Autodesk Inventor part; units mm, degrees
(part 4 of 10)
  spline S27 degree 5 poles (6.5254, -0.8339) (6.5255, -0.8339) (6.5256, -0.8339) (6.5259, -0.834) (6.5263, -0.834) (6.5268, -0.834) (6.5274, -0.8341) (6.5281, -0.8342) (6.5289, -0.8343) (6.5298, -0.8343) (6.5307, -0.8344) (6.5318, -0.8345) (6.5329, -0.8346) (6.5341, -0.8347) (6.5353, -0.8348) (6.5366, -0.8349) (6.5381, -0.8349) (6.5395, -0.835) (6.5411, -0.8351) (6.5427, -0.8352) (6.5444, -0.8353) (6.5462, -0.8354) (6.548, -0.8355) (6.55, -0.8356) (6.5519, -0.8356) (6.554, -0.8357) (6.5561, -0.8358) (6.5583, -0.8358) (6.5606, -0.8359) (6.5629, -0.8359) (6.5653, -0.836) (6.5678, -0.836) (6.5703, -0.836) (6.5729, -0.8361) (6.5755, -0.8361) (6.5788, -0.8361) (6.5821, -0.8361) (6.5856, -0.836) (6.5903, -0.836) (6.5964, -0.8359) (6.6022, -0.8358) (6.6081, -0.8356) (6.6149, -0.8353) (6.6206, -0.8351) (6.6249, -0.8349) (6.6293, -0.8347) (6.6352, -0.8344) (6.6406, -0.8341) (6.646, -0.8337) (6.6524, -0.8333) (6.6589, -0.8328) (6.6639, -0.8324) (6.6697, -0.832) (6.6757, -0.8314) (6.6809, -0.831) (6.6871, -0.8304) (6.6934, -0.8298) (6.6988, -0.8292) (6.7053, -0.8286) (6.7118, -0.8278) (6.7175, -0.8272) (6.7242, -0.8264) (6.731, -0.8256) (6.737, -0.8248) (6.7439, -0.8239) (6.751, -0.823) (6.7571, -0.8221) (6.7644, -0.8211) (6.7717, -0.82) (6.778, -0.8191) (6.7855, -0.8179) (6.7931, -0.8167) (6.7996, -0.8156) (6.8074, -0.8144) (6.8152, -0.813) (6.8219, -0.8118) (6.8299, -0.8104) (6.8379, -0.809) (6.8449, -0.8077) (6.8531, -0.8061) (6.8613, -0.8045) (6.8685, -0.8031) (6.8769, -0.8014) (6.8853, -0.7997) (6.8927, -0.7981) (6.9013, -0.7963) (6.91, -0.7944) (6.9175, -0.7927) (6.9263, -0.7907) (6.9352, -0.7887) (6.9428, -0.7869) (6.9519, -0.7848) (6.9609, -0.7826) (6.9688, -0.7806) (6.978, -0.7783) (6.9873, -0.776) (6.9953, -0.7739) (7.0047, -0.7715) (7.0142, -0.769) (7.0223, -0.7668) (7.0319, -0.7642) (7.0415, -0.7615) (7.0499, -0.7591) (7.0596, -0.7564) (7.0694, -0.7535) (7.0779, -0.7511) (7.0878, -0.7481) (7.0978, -0.7451) (7.1064, -0.7425) (7.1165, -0.7394) (7.1267, -0.7362) (7.1354, -0.7334) (7.1457, -0.7302) (7.156, -0.7268) (7.1649, -0.7239) (7.1753, -0.7205) (7.1857, -0.7169) (7.1947, -0.7139) (7.2053, -0.7103) (7.2159, -0.7066) (7.225, -0.7034) (7.2357, -0.6996) (7.2465, -0.6957) (7.2558, -0.6923) (7.2666, -0.6883) (7.2775, -0.6843) (7.2869, -0.6808) (7.2978, -0.6766) (7.3089, -0.6724) (7.3183, -0.6687) (7.3295, -0.6644) (7.3406, -0.66) (7.3502, -0.6561) (7.3614, -0.6516) (7.3727, -0.647) (7.3824, -0.643) (7.3937, -0.6383) (7.4051, -0.6335) (7.4149, -0.6294) (7.4264, -0.6245) (7.4379, -0.6195) (7.4478, -0.6152) (7.4594, -0.6101) (7.471, -0.605) (7.481, -0.6005) (7.4927, -0.5952) (7.5044, -0.5899) (7.5145, -0.5853) (7.5263, -0.5798) (7.5381, -0.5743) (7.5482, -0.5695) (7.5584, -0.5646) (7.5703, -0.5589) (7.5806, -0.554) (7.5908, -0.549) (7.6028, -0.5431) (7.6149, -0.5371) (7.6252, -0.5319) (7.6373, -0.5259) (7.6494, -0.5197) (7.6598, -0.5144) (7.6703, -0.509) (7.6842, -0.5017) (7.6964, -0.4953) (7.7087, -0.4888) (7.721, -0.4823) (7.7333, -0.4756) (7.7421, -0.4709) (7.7509, -0.4661) (7.7598, -0.4612) (7.7686, -0.4563) (7.7775, -0.4514) (7.7863, -0.4465) (7.7952, -0.4415) (7.8041, -0.4365) (7.813, -0.4314) (7.822, -0.4263) (7.8309, -0.4212) (7.8398, -0.4161) (7.8488, -0.4109) (7.8578, -0.4056) (7.8667, -0.4004) (7.8757, -0.3951) (7.8847, -0.3897) (7.8937, -0.3843) (7.9028, -0.3789) (7.9118, -0.3735) (7.9208, -0.368) (7.9299, -0.3625) (7.9389, -0.357) (7.9534, -0.348) (7.9662, -0.3401) (7.9771, -0.3333) (7.9862, -0.3275) (7.9935, -0.3229) knots 0 0 0 0 0 0 0.004167 0.008333 0.0125 0.016667 0.020833 0.025 0.029167 0.033333 0.0375 0.041667 0.045833 0.05 0.054167 0.058333 0.0625 0.066667 0.070833 0.075 0.079167 0.083333 0.0875 0.091667 0.095833 0.1 0.104167 0.108333 0.1125 0.116667 0.120833 0.125 0.129167 0.133333 0.1375 0.141667 0.15 0.154167 0.158333 0.170833 0.183333 0.1875 0.191667 0.2 0.204167 0.208333 0.2125 0.225 0.229167 0.233333 0.241667 0.245833 0.25 0.258333 0.2625 0.266667 0.275 0.279167 0.283333 0.291667 0.295833 0.3 0.308333 0.3125 0.316667 0.325 0.329167 0.333333 0.341667 0.345833 0.35 0.358333 0.3625 0.366667 0.375 0.379167 0.383333 0.391667 0.395833 0.4 0.408333 0.4125 0.416667 0.425 0.429167 0.433333 0.441667 0.445833 0.45 0.458333 0.4625 0.466667 0.475 0.479167 0.483333 0.491667 0.495833 0.5 0.508333 0.5125 0.516667 0.525 0.529167 0.533333 0.541667 0.545833 0.55 0.558333 0.5625 0.566667 0.575 0.579167 0.583333 0.591667 0.595833 0.6 0.608333 0.6125 0.616667 0.625 0.629167 0.633333 0.641667 0.645833 0.65 0.658333 0.6625 0.666667 0.675 0.679167 0.683333 0.691667 0.695833 0.7 0.708333 0.7125 0.716667 0.725 0.729167 0.733333 0.741667 0.745833 0.75 0.758333 0.7625 0.766667 0.775 0.779167 0.783333 0.791667 0.795833 0.8 0.804167 0.8125 0.816667 0.820833 0.829167 0.833333 0.8375 0.845833 0.85 0.854167 0.858333 0.870833 0.875 0.879167 0.883333 0.8875 0.891667 0.895833 0.9 0.904167 0.908333 0.9125 0.916667 0.920833 0.925 0.929167 0.933333 0.9375 0.941667 0.945833 0.95 0.954167 0.958333 0.9625 0.966667 0.970833 0.975 0.979167 0.983333 1 1 1 1 1 1
  line L55 (6.5248, 0.8338) -> (5.7036, 0.7289)
  point P0 (0, 0)
sketch "Block2" plane through (0, 0, 0) normal (0, 0, 1) x (1, 0, 0)
  arc A0 (-0.6063, 1.979) -> (-0.252, 3.0198) centre (-4.8955, 4.02) ccw
  line L0 (0.1956, 1.5974) -> (-0.6063, 1.979)
  line L1 (0.1962, 1.5971) -> (0.1956, 1.5974)
  spline S0 degree 5 poles (1.0882, 0.3875) (1.0858, 0.3933) (1.0826, 0.401) (1.0786, 0.4107) (1.0738, 0.4222) (1.0681, 0.4355) (1.064, 0.4451) (1.0599, 0.4545) (1.0558, 0.464) (1.0517, 0.4734) (1.0476, 0.4827) (1.0434, 0.4921) (1.0393, 0.5014) (1.0351, 0.5106) (1.0309, 0.5199) (1.0267, 0.5291) (1.0225, 0.5382) (1.0183, 0.5474) (1.0141, 0.5565) (1.0098, 0.5655) (1.0056, 0.5745) (1.0013, 0.5835) (0.997, 0.5925) (0.9928, 0.6014) (0.9885, 0.6103) (0.9841, 0.6191) (0.9798, 0.6279) (0.9755, 0.6367) (0.9711, 0.6454) (0.9668, 0.6541) (0.9616, 0.6645) (0.9563, 0.6748) (0.951, 0.6851) (0.9449, 0.6971) (0.9387, 0.7089) (0.9334, 0.719) (0.9281, 0.7291) (0.9227, 0.7391) (0.9174, 0.7491) (0.912, 0.759) (0.9067, 0.7688) (0.9004, 0.7802) (0.8941, 0.7916) (0.8887, 0.8012) (0.8824, 0.8125) (0.876, 0.8236) (0.8706, 0.8331) (0.8642, 0.8441) (0.8579, 0.855) (0.8524, 0.8643) (0.8451, 0.8766) (0.8378, 0.8889) (0.8314, 0.8995) (0.8249, 0.91) (0.8167, 0.9234) (0.8102, 0.9338) (0.8038, 0.9441) (0.7973, 0.9543) (0.789, 0.9673) (0.7826, 0.9774) (0.7761, 0.9874) (0.7687, 0.9987) (0.7613, 1.0098) (0.7557, 1.0182) (0.7492, 1.0278) (0.7428, 1.0374) (0.7372, 1.0455) (0.7307, 1.055) (0.7242, 1.0643) (0.7187, 1.0723) (0.7122, 1.0815) (0.7057, 1.0906) (0.7001, 1.0983) (0.6936, 1.1073) (0.6872, 1.1162) (0.6816, 1.1238) (0.6752, 1.1326) (0.6687, 1.1412) (0.6632, 1.1486) (0.6567, 1.1571) (0.6503, 1.1656) (0.6447, 1.1727) (0.6383, 1.1811) (0.6319, 1.1893) (0.6264, 1.1963) (0.62, 1.2043) (0.6136, 1.2123) (0.6081, 1.2191) (0.6018, 1.2269) (0.5954, 1.2347) (0.59, 1.2413) (0.5837, 1.2489) (0.5774, 1.2564) (0.572, 1.2628) (0.5657, 1.2702) (0.5594, 1.2775) (0.5541, 1.2837) (0.5479, 1.2908) (0.5416, 1.2979) (0.5363, 1.3039) (0.5302, 1.3108) (0.524, 1.3176) (0.5188, 1.3234) (0.5127, 1.3301) (0.5066, 1.3367) (0.5014, 1.3423) (0.4954, 1.3487) (0.4894, 1.3551) (0.4843, 1.3605) (0.4783, 1.3667) (0.4724, 1.3728) (0.4673, 1.378) (0.4615, 1.384) (0.4557, 1.3898) (0.4507, 1.3948) (0.4449, 1.4006) (0.4392, 1.4062) (0.4343, 1.411) (0.4286, 1.4165) (0.423, 1.4219) (0.4182, 1.4265) (0.4127, 1.4317) (0.4071, 1.4369) (0.4024, 1.4413) (0.397, 1.4463) (0.3916, 1.4512) (0.387, 1.4554) (0.3817, 1.4602) (0.3764, 1.4649) (0.372, 1.4689) (0.3668, 1.4734) (0.3617, 1.4779) (0.3573, 1.4816) (0.3523, 1.4859) (0.3473, 1.4901) (0.3431, 1.4937) (0.3382, 1.4978) (0.3333, 1.5018) (0.3293, 1.5051) (0.3245, 1.5089) (0.3199, 1.5127) (0.3159, 1.5158) (0.3114, 1.5194) (0.3069, 1.5229) (0.3031, 1.5259) (0.2988, 1.5292) (0.2945, 1.5325) (0.2908, 1.5353) (0.2867, 1.5384) (0.2826, 1.5414) (0.2791, 1.5439) (0.2752, 1.5468) (0.2713, 1.5496) (0.268, 1.552) (0.2648, 1.5542) (0.2606, 1.5572) (0.257, 1.5597) (0.253, 1.5624) (0.2491, 1.5651) (0.2453, 1.5676) (0.2426, 1.5694) (0.2399, 1.5712) (0.2377, 1.5726) (0.2356, 1.574) (0.2335, 1.5753) (0.2314, 1.5766) (0.2294, 1.5779) (0.2275, 1.5791) (0.2256, 1.5803) (0.2237, 1.5814) (0.2219, 1.5825) (0.2202, 1.5836) (0.2185, 1.5846) (0.2168, 1.5856) (0.2153, 1.5865) (0.2137, 1.5874) (0.2123, 1.5883) (0.2108, 1.5891) (0.2095, 1.5899) (0.2082, 1.5906) (0.2069, 1.5913) (0.2057, 1.592) (0.2046, 1.5926) (0.2036, 1.5932) (0.2026, 1.5938) (0.2016, 1.5943) (0.2008, 1.5947) (0.1999, 1.5952) (0.1992, 1.5955) (0.1985, 1.5959) (0.1979, 1.5962) (0.1973, 1.5965) (0.1968, 1.5968) (0.1965, 1.5969) (0.1963, 1.597) (0.1962, 1.5971) knots -1 -1 -1 -1 -1 -1 -0.9875 -0.983333 -0.979167 -0.975 -0.970833 -0.966667 -0.9625 -0.958333 -0.954167 -0.95 -0.945833 -0.941667 -0.9375 -0.933333 -0.929167 -0.925 -0.920833 -0.916667 -0.9125 -0.908333 -0.904167 -0.9 -0.895833 -0.891667 -0.8875 -0.883333 -0.879167 -0.875 -0.870833 -0.8625 -0.858333 -0.854167 -0.845833 -0.841667 -0.8375 -0.833333 -0.829167 -0.820833 -0.816667 -0.8125 -0.804167 -0.8 -0.795833 -0.7875 -0.783333 -0.779167 -0.770833 -0.766667 -0.7625 -0.75 -0.745833 -0.741667 -0.7375 -0.725 -0.720833 -0.716667 -0.7125 -0.7 -0.695833 -0.691667 -0.683333 -0.679167 -0.675 -0.666667 -0.6625 -0.658333 -0.65 -0.645833 -0.641667 -0.633333 -0.629167 -0.625 -0.616667 -0.6125 -0.608333 -0.6 -0.595833 -0.591667 -0.583333 -0.579167 -0.575 -0.566667 -0.5625 -0.558333 -0.55 -0.545833 -0.541667 -0.533333 -0.529167 -0.525 -0.516667 -0.5125 -0.508333 -0.5 -0.495833 -0.491667 -0.483333 -0.479167 -0.475 -0.466667 -0.4625 -0.458333 -0.45 -0.445833 -0.441667 -0.433333 -0.429167 -0.425 -0.416667 -0.4125 -0.408333 -0.4 -0.395833 -0.391667 -0.383333 -0.379167 -0.375 -0.366667 -0.3625 -0.358333 -0.35 -0.345833 -0.341667 -0.333333 -0.329167 -0.325 -0.316667 -0.3125 -0.308333 -0.3 -0.295833 -0.291667 -0.283333 -0.279167 -0.275 -0.266667 -0.2625 -0.258333 -0.25 -0.245833 -0.241667 -0.233333 -0.229167 -0.225 -0.216667 -0.2125 -0.208333 -0.2 -0.195833 -0.191667 -0.183333 -0.179167 -0.175 -0.170833 -0.158333 -0.154167 -0.145833 -0.141667 -0.1375 -0.133333 -0.129167 -0.125 -0.120833 -0.116667 -0.1125 -0.108333 -0.104167 -0.1 -0.095833 -0.091667 -0.0875 -0.083333 -0.079167 -0.075 -0.070833 -0.066667 -0.0625 -0.058333 -0.054167 -0.05 -0.045833 -0.041667 -0.0375 -0.033333 -0.029167 -0.025 -0.020833 -0.016667 -0.0125 -0.008333 0 0 0 0 0 0
  arc A1 (0.7429, -0.1283) -> (1.0882, 0.3875) centre (-4.8955, 4.02) ccw
  line L2 (-0.7158, 0.236) -> (-0.7153, 0.2355)
  spline S1 degree 5 poles (-0.7153, 0.2355) (-0.7153, 0.2355) (-0.7152, 0.2354) (-0.715, 0.2353) (-0.7147, 0.235) (-0.7143, 0.2347) (-0.7139, 0.2343) (-0.7133, 0.2338) (-0.7128, 0.2334) (-0.7121, 0.2328) (-0.7114, 0.2322) (-0.7106, 0.2316) (-0.7098, 0.2309) (-0.7089, 0.2302) (-0.708, 0.2295) (-0.707, 0.2287) (-0.7059, 0.2278) (-0.7048, 0.2269) (-0.7036, 0.226) (-0.7024, 0.2251) (-0.7011, 0.2241) (-0.6997, 0.223) (-0.6983, 0.2219) (-0.6968, 0.2208) (-0.6953, 0.2197) (-0.6937, 0.2185) (-0.6921, 0.2173) (-0.6904, 0.2161) (-0.6886, 0.2148) (-0.6868, 0.2135) (-0.6849, 0.2121) (-0.683, 0.2108) (-0.6806, 0.2091) (-0.6781, 0.2074) (-0.6756, 0.2056) (-0.6725, 0.2035) (-0.6693, 0.2014) (-0.6665, 0.1995) (-0.6631, 0.1972) (-0.6596, 0.1949) (-0.6565, 0.1929) (-0.6534, 0.1909) (-0.6496, 0.1885) (-0.6446, 0.1853) (-0.6394, 0.1821) (-0.634, 0.1788) (-0.6285, 0.1754) (-0.6227, 0.172) (-0.6182, 0.1693) (-0.6135, 0.1666) (-0.6088, 0.1638) (-0.6032, 0.1606) (-0.5982, 0.1578) (-0.5938, 0.1554) (-0.5887, 0.1525) (-0.5834, 0.1497) (-0.5788, 0.1472) (-0.5734, 0.1442) (-0.5678, 0.1413) (-0.563, 0.1387) (-0.5572, 0.1358) (-0.5514, 0.1328) (-0.5463, 0.1302) (-0.5403, 0.1271) (-0.5342, 0.1241) (-0.5289, 0.1215) (-0.5226, 0.1184) (-0.5162, 0.1153) (-0.5107, 0.1127) (-0.5041, 0.1096) (-0.4975, 0.1065) (-0.4917, 0.1038) (-0.4849, 0.1007) (-0.478, 0.0975) (-0.472, 0.0949) (-0.4649, 0.0917) (-0.4577, 0.0886) (-0.4515, 0.0859) (-0.4442, 0.0827) (-0.4367, 0.0796) (-0.4303, 0.0769) (-0.4227, 0.0737) (-0.415, 0.0706) (-0.4083, 0.0679) (-0.4005, 0.0647) (-0.3925, 0.0616) (-0.3856, 0.0589) (-0.3775, 0.0558) (-0.3693, 0.0527) (-0.3623, 0.05) (-0.3539, 0.0469) (-0.3455, 0.0438) (-0.3382, 0.0411) (-0.3296, 0.038) (-0.3209, 0.035) (-0.3134, 0.0323) (-0.3045, 0.0293) (-0.2956, 0.0262) (-0.2879, 0.0237) (-0.2788, 0.0206) (-0.2697, 0.0176) (-0.2618, 0.0151) (-0.2525, 0.0121) (-0.2431, 0.0091) (-0.235, 0.0066) (-0.2254, 0.0037) (-0.2158, 0.0008) (-0.2075, -0.0017) (-0.1977, -0.0046) (-0.1879, -0.0074) (-0.1794, -0.0099) (-0.1694, -0.0127) (-0.1593, -0.0155) (-0.1506, -0.0179) (-0.1404, -0.0206) (-0.1301, -0.0234) (-0.1213, -0.0257) (-0.1108, -0.0284) (-0.1003, -0.031) (-0.0913, -0.0333) (-0.0806, -0.0359) (-0.0699, -0.0385) (-0.0606, -0.0407) (-0.0498, -0.0432) (-0.0389, -0.0457) (-0.0294, -0.0479) (-0.0184, -0.0503) (-0.0072, -0.0528) (0.0024, -0.0548) (0.0136, -0.0572) (0.025, -0.0595) (0.0347, -0.0615) (0.0462, -0.0638) (0.0578, -0.0661) (0.0677, -0.068) (0.0794, -0.0701) (0.0911, -0.0723) (0.1012, -0.0741) (0.1131, -0.0762) (0.125, -0.0783) (0.1353, -0.08) (0.1474, -0.082) (0.1595, -0.084) (0.1699, -0.0856) (0.1822, -0.0875) (0.1945, -0.0894) (0.2051, -0.0909) (0.2193, -0.0929) (0.2336, -0.0949) (0.2462, -0.0966) (0.2589, -0.0983) (0.2716, -0.0999) (0.2862, -0.1017) (0.3008, -0.1034) (0.3156, -0.1051) (0.3305, -0.1067) (0.3473, -0.1085) (0.3585, -0.1096) (0.3698, -0.1108) (0.3849, -0.1122) (0.4002, -0.1136) (0.4135, -0.1147) (0.427, -0.1158) (0.4405, -0.1169) (0.4501, -0.1176) (0.4598, -0.1183) (0.4696, -0.119) (0.4793, -0.1197) (0.4891, -0.1203) (0.4989, -0.1209) (0.5088, -0.1215) (0.5187, -0.1221) (0.5286, -0.1226) (0.5385, -0.1232) (0.5485, -0.1237) (0.5584, -0.1241) (0.5685, -0.1246) (0.5785, -0.125) (0.5886, -0.1254) (0.5987, -0.1258) (0.6088, -0.1261) (0.619, -0.1264) (0.6291, -0.1267) (0.6394, -0.127) (0.6496, -0.1272) (0.6599, -0.1275) (0.6701, -0.1277) (0.6805, -0.1278) (0.6908, -0.128) (0.7053, -0.1281) (0.7178, -0.1282) (0.7283, -0.1283) (0.7366, -0.1283) (0.7429, -0.1283) knots 0 0 0 0 0 0 0.004167 0.008333 0.0125 0.016667 0.020833 0.025 0.029167 0.033333 0.0375 0.041667 0.045833 0.05 0.054167 0.058333 0.0625 0.066667 0.070833 0.075 0.079167 0.083333 0.0875 0.091667 0.095833 0.1 0.104167 0.108333 0.1125 0.116667 0.120833 0.125 0.129167 0.1375 0.141667 0.145833 0.154167 0.158333 0.1625 0.170833 0.175 0.179167 0.183333 0.191667 0.208333 0.2125 0.216667 0.220833 0.229167 0.2375 0.241667 0.245833 0.254167 0.258333 0.2625 0.270833 0.275 0.279167 0.2875 0.291667 0.295833 0.304167 0.308333 0.3125 0.320833 0.325 0.329167 0.3375 0.341667 0.345833 0.354167 0.358333 0.3625 0.370833 0.375 0.379167 0.3875 0.391667 0.395833 0.404167 0.408333 0.4125 0.420833 0.425 0.429167 0.4375 0.441667 0.445833 0.454167 0.458333 0.4625 0.470833 0.475 0.479167 0.4875 0.491667 0.495833 0.504167 0.508333 0.5125 0.520833 0.525 0.529167 0.5375 0.541667 0.545833 0.554167 0.558333 0.5625 0.570833 0.575 0.579167 0.5875 0.591667 0.595833 0.604167 0.608333 0.6125 0.620833 0.625 0.629167 0.6375 0.641667 0.645833 0.654167 0.658333 0.6625 0.670833 0.675 0.679167 0.6875 0.691667 0.695833 0.704167 0.708333 0.7125 0.720833 0.725 0.729167 0.7375 0.741667 0.745833 0.754167 0.758333 0.7625 0.770833 0.775 0.779167 0.791667 0.795833 0.8 0.804167 0.808333 0.825 0.829167 0.833333 0.8375 0.845833 0.85 0.854167 0.866667 0.870833 0.875 0.879167 0.883333 0.8875 0.891667 0.895833 0.9 0.904167 0.908333 0.9125 0.916667 0.920833 0.925 0.929167 0.933333 0.9375 0.941667 0.945833 0.95 0.954167 0.958333 0.9625 0.966667 0.970833 0.975 0.979167 0.983333 0.9875 1 1 1 1 1 1
  line L3 (-1.3742, 0.832) -> (-0.7158, 0.236)
  arc A2 (-2.2015, 0.1079) -> (-1.3742, 0.832) centre (-4.8955, 4.02) ccw
  line L4 (0.6162, 2.8328) -> (0.6169, 2.8327)
  line L5 (-0.252, 3.0198) -> (0.6162, 2.8328)
  spline S2 degree 5 poles (0.6169, 2.8327) (0.6169, 2.8326) (0.6171, 2.8326) (0.6173, 2.8326) (0.6176, 2.8325) (0.6182, 2.8324) (0.6188, 2.8323) (0.6194, 2.8322) (0.6202, 2.832) (0.621, 2.8319) (0.6219, 2.8317) (0.6229, 2.8316) (0.6239, 2.8314) (0.6251, 2.8312) (0.6263, 2.831) (0.6275, 2.8309) (0.6289, 2.8307) (0.6303, 2.8305) (0.6318, 2.8302) (0.6333, 2.83) (0.6349, 2.8298) (0.6366, 2.8296) (0.6384, 2.8294) (0.6402, 2.8292) (0.6421, 2.8289) (0.6441, 2.8287) (0.6461, 2.8285) (0.6482, 2.8283) (0.6504, 2.828) (0.6526, 2.8278) (0.6549, 2.8276) (0.6572, 2.8274) (0.6601, 2.8271) (0.6631, 2.8269) (0.6662, 2.8266) (0.67, 2.8263) (0.6738, 2.826) (0.6772, 2.8258) (0.6812, 2.8256) (0.6854, 2.8253) (0.6891, 2.8251) (0.6935, 2.8249) (0.698, 2.8247) (0.7019, 2.8246) (0.7066, 2.8244) (0.7115, 2.8243) (0.7157, 2.8241) (0.7207, 2.824) (0.7258, 2.824) (0.7303, 2.8239) (0.7356, 2.8239) (0.7411, 2.8238) (0.7458, 2.8238) (0.7514, 2.8239) (0.7572, 2.8239) (0.7621, 2.824) (0.768, 2.8241) (0.774, 2.8242) (0.7793, 2.8244) (0.7855, 2.8246) (0.7917, 2.8248) (0.7972, 2.825) (0.8037, 2.8253) (0.8102, 2.8256) (0.8159, 2.8259) (0.8226, 2.8263) (0.8294, 2.8267) (0.8353, 2.8271) (0.8423, 2.8276) (0.8494, 2.8281) (0.8555, 2.8286) (0.8627, 2.8291) (0.87, 2.8298) (0.8764, 2.8304) (0.8839, 2.8311) (0.8914, 2.8318) (0.8979, 2.8325) (0.9056, 2.8333) (0.9134, 2.8342) (0.9202, 2.8349) (0.9281, 2.8359) (0.9361, 2.8369) (0.9431, 2.8378) (0.9512, 2.8388) (0.9594, 2.84) (0.9666, 2.841) (0.9749, 2.8422) (0.9834, 2.8434) (0.9907, 2.8445) (0.9993, 2.8459) (1.0079, 2.8473) (1.0154, 2.8485) (1.0242, 2.85) (1.033, 2.8515) (1.0407, 2.8529) (1.0497, 2.8545) (1.0587, 2.8562) (1.0666, 2.8577) (1.0757, 2.8594) (1.085, 2.8612) (1.093, 2.8629) (1.1023, 2.8648) (1.1118, 2.8668) (1.1199, 2.8685) (1.1294, 2.8706) (1.1391, 2.8727) (1.1473, 2.8746) (1.1571, 2.8768) (1.1668, 2.8791) (1.1753, 2.8811) (1.1852, 2.8835) (1.1951, 2.8859) (1.2037, 2.8881) (1.2138, 2.8906) (1.2239, 2.8932) (1.2326, 2.8955) (1.2428, 2.8983) (1.2531, 2.901) (1.2619, 2.9035) (1.2723, 2.9063) (1.2828, 2.9093) (1.2917, 2.9119) (1.3023, 2.9149) (1.3128, 2.918) (1.3219, 2.9208) (1.3326, 2.924) (1.3433, 2.9273) (1.3526, 2.9301) (1.3634, 2.9335) (1.3742, 2.937) (1.3836, 2.94) (1.3945, 2.9436) (1.4055, 2.9473) (1.415, 2.9504) (1.426, 2.9542) (1.4372, 2.958) (1.4467, 2.9613) (1.4579, 2.9653) (1.4692, 2.9693) (1.4789, 2.9727) (1.4902, 2.9769) (1.5015, 2.9811) (1.5113, 2.9847) (1.5228, 2.989) (1.5342, 2.9934) (1.5441, 2.9972) (1.5557, 3.0016) (1.5672, 3.0062) (1.5772, 3.0102) (1.5872, 3.0142) (1.6022, 3.0202) (1.6157, 3.0257) (1.6291, 3.0313) (1.6426, 3.037) (1.6596, 3.0443) (1.6715, 3.0494) (1.6834, 3.0546) (1.6954, 3.0599) (1.7108, 3.0668) (1.7229, 3.0722) (1.7349, 3.0777) (1.7488, 3.084) (1.7627, 3.0905) (1.7731, 3.0954) (1.7835, 3.1003) (1.794, 3.1053) (1.8028, 3.1095) (1.8115, 3.1138) (1.8203, 3.118) (1.8291, 3.1223) (1.8379, 3.1267) (1.8467, 3.1311) (1.8555, 3.1355) (1.8643, 3.1399) (1.8732, 3.1444) (1.882, 3.1489) (1.8909, 3.1535) (1.8998, 3.1581) (1.9087, 3.1627) (1.9176, 3.1673) (1.9265, 3.172) (1.9355, 3.1768) (1.9444, 3.1815) (1.9534, 3.1863) (1.9623, 3.1911) (1.9713, 3.196) (1.9803, 3.2009) (1.9893, 3.2059) (1.9983, 3.2108) (2.0073, 3.2159) (2.0164, 3.2209) (2.029, 3.228) (2.0399, 3.2342) (2.0489, 3.2394) (2.0562, 3.2435) (2.0617, 3.2467) knots 0 0 0 0 0 0 0.004167 0.008333 0.0125 0.016667 0.020833 0.025 0.029167 0.033333 0.0375 0.041667 0.045833 0.05 0.054167 0.058333 0.0625 0.066667 0.070833 0.075 0.079167 0.083333 0.0875 0.091667 0.095833 0.1 0.104167 0.108333 0.1125 0.116667 0.120833 0.125 0.129167 0.1375 0.141667 0.145833 0.154167 0.158333 0.1625 0.170833 0.175 0.179167 0.1875 0.191667 0.195833 0.204167 0.208333 0.2125 0.220833 0.225 0.229167 0.2375 0.241667 0.245833 0.254167 0.258333 0.2625 0.270833 0.275 0.279167 0.2875 0.291667 0.295833 0.304167 0.308333 0.3125 0.320833 0.325 0.329167 0.3375 0.341667 0.345833 0.354167 0.358333 0.3625 0.370833 0.375 0.379167 0.3875 0.391667 0.395833 0.404167 0.408333 0.4125 0.420833 0.425 0.429167 0.4375 0.441667 0.445833 0.454167 0.458333 0.4625 0.470833 0.475 0.479167 0.4875 0.491667 0.495833 0.504167 0.508333 0.5125 0.520833 0.525 0.529167 0.5375 0.541667 0.545833 0.554167 0.558333 0.5625 0.570833 0.575 0.579167 0.5875 0.591667 0.595833 0.604167 0.608333 0.6125 0.620833 0.625 0.629167 0.6375 0.641667 0.645833 0.654167 0.658333 0.6625 0.670833 0.675 0.679167 0.6875 0.691667 0.695833 0.704167 0.708333 0.7125 0.720833 0.725 0.729167 0.7375 0.741667 0.745833 0.754167 0.758333 0.7625 0.770833 0.775 0.779167 0.783333 0.8 0.804167 0.808333 0.8125 0.825 0.829167 0.833333 0.8375 0.85 0.854167 0.858333 0.866667 0.870833 0.875 0.879167 0.883333 0.8875 0.891667 0.895833 0.9 0.904167 0.908333 0.9125 0.916667 0.920833 0.925 0.929167 0.933333 0.9375 0.941667 0.945833 0.95 0.954167 0.958333 0.9625 0.966667 0.970833 0.975 0.979167 0.983333 0.9875 1 1 1 1 1 1
  line L6 (0.7249, 4.4675) -> (-0.1605, 4.397)
  line L7 (0.7255, 4.4675) -> (0.7249, 4.4675)
  arc A3 (-0.1605, 4.397) -> (-0.374, 5.4756) centre (-4.8955, 4.02) ccw
  spline S3 degree 5 poles (2.1028, 3.866) (2.0978, 3.8698) (2.0912, 3.8749) (2.0829, 3.8813) (2.0729, 3.8888) (2.0613, 3.8976) (2.053, 3.9038) (2.0448, 3.9099) (2.0365, 3.916) (2.0282, 3.9221) (2.02, 3.9282) (2.0117, 3.9342) (2.0035, 3.9402) (1.9952, 3.9461) (1.987, 3.952) (1.9788, 3.9579) (1.9705, 3.9637) (1.9623, 3.9695) (1.9541, 3.9753) (1.9459, 3.981) (1.9377, 3.9867) (1.9295, 3.9923) (1.9213, 3.9979) (1.9132, 4.0035) (1.905, 4.0091) (1.8969, 4.0146) (1.8887, 4.02) (1.8806, 4.0255) (1.8724, 4.0308) (1.8643, 4.0362) (1.8546, 4.0426) (1.8449, 4.0489) (1.8352, 4.0552) (1.8239, 4.0625) (1.8126, 4.0696) (1.8029, 4.0757) (1.7933, 4.0818) (1.7837, 4.0878) (1.7741, 4.0937) (1.7645, 4.0996) (1.7549, 4.1055) (1.7438, 4.1122) (1.7326, 4.1189) (1.7231, 4.1246) (1.712, 4.1311) (1.701, 4.1376) (1.6915, 4.1431) (1.6805, 4.1494) (1.6696, 4.1557) (1.6602, 4.161) (1.6492, 4.1672) (1.6383, 4.1733) (1.629, 4.1784) (1.6166, 4.1852) (1.6043, 4.1919) (1.5935, 4.1977) (1.5828, 4.2034) (1.569, 4.2107) (1.5583, 4.2162) (1.5477, 4.2217) (1.5371, 4.2271) (1.5235, 4.234) (1.513, 4.2393) (1.5025, 4.2445) (1.4906, 4.2504) (1.4787, 4.2561) (1.4698, 4.2604) (1.4594, 4.2653) (1.4492, 4.2702) (1.4404, 4.2743) (1.4301, 4.279) (1.42, 4.2836) (1.4113, 4.2876) (1.4012, 4.2921) (1.3911, 4.2966) (1.3825, 4.3004) (1.3725, 4.3047) (1.3626, 4.309) (1.3541, 4.3126) (1.3443, 4.3168) (1.3345, 4.3209) (1.3261, 4.3243) (1.3164, 4.3283) (1.3067, 4.3322) (1.2985, 4.3355) (1.2889, 4.3393) (1.2794, 4.343) (1.2712, 4.3462) (1.2618, 4.3498) (1.2524, 4.3533) (1.2444, 4.3563) (1.2351, 4.3597) (1.2259, 4.3631) (1.2181, 4.3659) (1.2089, 4.3692) (1.1999, 4.3724) (1.1921, 4.3751) (1.1832, 4.3781) (1.1743, 4.3812) (1.1667, 4.3837) (1.1579, 4.3866) (1.1491, 4.3894) (1.1417, 4.3918) (1.1331, 4.3946) (1.1245, 4.3972) (1.1172, 4.3995) (1.1088, 4.4021) (1.1004, 4.4046) (1.0933, 4.4067) (1.085, 4.4091) (1.0768, 4.4114) (1.0699, 4.4134) (1.0618, 4.4156) (1.0538, 4.4178) (1.047, 4.4196) (1.0391, 4.4217) (1.0314, 4.4237) (1.0247, 4.4254) (1.0171, 4.4274) (1.0095, 4.4292) (1.0031, 4.4308) (0.9956, 4.4326) (0.9883, 4.4343) (0.982, 4.4357) (0.9748, 4.4374) (0.9676, 4.4389) (0.9616, 4.4403) (0.9546, 4.4417) (0.9477, 4.4432) (0.9418, 4.4444) (0.9351, 4.4457) (0.9284, 4.447) (0.9227, 4.4481) (0.9162, 4.4493) (0.9098, 4.4505) (0.9044, 4.4514) (0.8981, 4.4525) (0.8919, 4.4536) (0.8867, 4.4544) (0.8807, 4.4554) (0.8748, 4.4563) (0.8698, 4.457) (0.8641, 4.4579) (0.8584, 4.4587) (0.8537, 4.4593) (0.8482, 4.4601) (0.8429, 4.4608) (0.8384, 4.4613) (0.8332, 4.4619) (0.8281, 4.4625) (0.8239, 4.463) (0.819, 4.4635) (0.8142, 4.464) (0.8102, 4.4644) (0.8063, 4.4647) (0.8012, 4.4652) (0.7968, 4.4656) (0.792, 4.4659) (0.7873, 4.4663) (0.7828, 4.4666) (0.7795, 4.4668) (0.7763, 4.467) (0.7737, 4.4671) (0.7711, 4.4672) (0.7686, 4.4673) (0.7662, 4.4674) (0.7639, 4.4675) (0.7616, 4.4676) (0.7593, 4.4677) (0.7571, 4.4678) (0.755, 4.4678) (0.753, 4.4679) (0.751, 4.4679) (0.7491, 4.4679) (0.7473, 4.4679) (0.7455, 4.468) (0.7438, 4.468) (0.7421, 4.468) (0.7406, 4.468) (0.7391, 4.468) (0.7377, 4.4679) (0.7363, 4.4679) (0.735, 4.4679) (0.7338, 4.4679) (0.7327, 4.4678) (0.7316, 4.4678) (0.7306, 4.4678) (0.7297, 4.4677) (0.7289, 4.4677) (0.7281, 4.4677) (0.7274, 4.4676) (0.7267, 4.4676) (0.7262, 4.4676) (0.7259, 4.4676) (0.7256, 4.4676) (0.7255, 4.4675) knots -1 -1 -1 -1 -1 -1 -0.9875 -0.983333 -0.979167 -0.975 -0.970833 -0.966667 -0.9625 -0.958333 -0.954167 -0.95 -0.945833 -0.941667 -0.9375 -0.933333 -0.929167 -0.925 -0.920833 -0.916667 -0.9125 -0.908333 -0.904167 -0.9 -0.895833 -0.891667 -0.8875 -0.883333 -0.879167 -0.875 -0.870833 -0.8625 -0.858333 -0.854167 -0.845833 -0.841667 -0.8375 -0.833333 -0.829167 -0.820833 -0.816667 -0.8125 -0.804167 -0.8 -0.795833 -0.7875 -0.783333 -0.779167 -0.770833 -0.766667 -0.7625 -0.754167 -0.75 -0.745833 -0.733333 -0.729167 -0.725 -0.720833 -0.708333 -0.704167 -0.7 -0.695833 -0.683333 -0.679167 -0.675 -0.666667 -0.6625 -0.658333 -0.65 -0.645833 -0.641667 -0.633333 -0.629167 -0.625 -0.616667 -0.6125 -0.608333 -0.6 -0.595833 -0.591667 -0.583333 -0.579167 -0.575 -0.566667 -0.5625 -0.558333 -0.55 -0.545833 -0.541667 -0.533333 -0.529167 -0.525 -0.516667 -0.5125 -0.508333 -0.5 -0.495833 -0.491667 -0.483333 -0.479167 -0.475 -0.466667 -0.4625 -0.458333 -0.45 -0.445833 -0.441667 -0.433333 -0.429167 -0.425 -0.416667 -0.4125 -0.408333 -0.4 -0.395833 -0.391667 -0.383333 -0.379167 -0.375 -0.366667 -0.3625 -0.358333 -0.35 -0.345833 -0.341667 -0.333333 -0.329167 -0.325 -0.316667 -0.3125 -0.308333 -0.3 -0.295833 -0.291667 -0.283333 -0.279167 -0.275 -0.266667 -0.2625 -0.258333 -0.25 -0.245833 -0.241667 -0.233333 -0.229167 -0.225 -0.216667 -0.2125 -0.208333 -0.2 -0.195833 -0.191667 -0.183333 -0.179167 -0.175 -0.170833 -0.158333 -0.154167 -0.145833 -0.141667 -0.1375 -0.133333 -0.129167 -0.125 -0.120833 -0.116667 -0.1125 -0.108333 -0.104167 -0.1 -0.095833 -0.091667 -0.0875 -0.083333 -0.079167 -0.075 -0.070833 -0.066667 -0.0625 -0.058333 -0.054167 -0.05 -0.045833 -0.041667 -0.0375 -0.033333 -0.029167 -0.025 -0.020833 -0.016667 -0.0125 -0.008333 0 0 0 0 0 0
  arc A4 (2.0617, 3.2467) -> (2.1028, 3.866) centre (-4.8955, 4.02) ccw
  line L8 (-10.4072, 5.2072) -> (-10.4079, 5.2073)
  line L9 (-9.539, 5.0202) -> (-10.4072, 5.2072)
  spline S4 degree 5 poles (-10.4079, 5.2073) (-10.4079, 5.2073) (-10.4081, 5.2073) (-10.4083, 5.2074) (-10.4086, 5.2075) (-10.4092, 5.2076) (-10.4098, 5.2077) (-10.4104, 5.2078) (-10.4112, 5.2079) (-10.412, 5.2081) (-10.4129, 5.2082) (-10.4139, 5.2084) (-10.4149, 5.2086) (-10.4161, 5.2087) (-10.4173, 5.2089) (-10.4185, 5.2091) (-10.4199, 5.2093) (-10.4213, 5.2095) (-10.4228, 5.2097) (-10.4243, 5.2099) (-10.4259, 5.2101) (-10.4276, 5.2104) (-10.4294, 5.2106) (-10.4312, 5.2108) (-10.4331, 5.211) (-10.4351, 5.2113) (-10.4371, 5.2115) (-10.4392, 5.2117) (-10.4414, 5.2119) (-10.4436, 5.2122) (-10.4459, 5.2124) (-10.4482, 5.2126) (-10.4511, 5.2129) (-10.4541, 5.2131) (-10.4572, 5.2134) (-10.461, 5.2136) (-10.4648, 5.2139) (-10.4682, 5.2141) (-10.4722, 5.2144) (-10.4764, 5.2146) (-10.4801, 5.2148) (-10.4845, 5.215) (-10.489, 5.2152) (-10.4929, 5.2154) (-10.4976, 5.2156) (-10.5025, 5.2157) (-10.5067, 5.2158) (-10.5117, 5.2159) (-10.5168, 5.216) (-10.5213, 5.2161) (-10.5266, 5.2161) (-10.5321, 5.2161) (-10.5368, 5.2161) (-10.5424, 5.2161) (-10.5482, 5.2161) (-10.5531, 5.216) (-10.559, 5.2159) (-10.565, 5.2157) (-10.5703, 5.2156) (-10.5765, 5.2154) (-10.5827, 5.2152) (-10.5882, 5.215) (-10.5947, 5.2147) (-10.6012, 5.2144) (-10.6069, 5.2141) (-10.6136, 5.2137) (-10.6204, 5.2133) (-10.6263, 5.2129) (-10.6333, 5.2124) (-10.6404, 5.2119) (-10.6465, 5.2114) (-10.6537, 5.2108) (-10.661, 5.2102) (-10.6674, 5.2096) (-10.6749, 5.2089) (-10.6824, 5.2082) (-10.6889, 5.2075) (-10.6966, 5.2067) (-10.7044, 5.2058) (-10.7112, 5.205) (-10.7191, 5.2041) (-10.7271, 5.2031) (-10.7341, 5.2022) (-10.7422, 5.2011) (-10.7504, 5.2) (-10.7576, 5.199) (-10.7659, 5.1978) (-10.7744, 5.1965) (-10.7817, 5.1954) (-10.7903, 5.1941) (-10.7989, 5.1927) (-10.8064, 5.1915) (-10.8152, 5.19) (-10.824, 5.1885) (-10.8317, 5.1871) (-10.8407, 5.1855) (-10.8497, 5.1838) (-10.8576, 5.1823) (-10.8667, 5.1805) (-10.876, 5.1787) (-10.884, 5.1771) (-10.8933, 5.1752) (-10.9028, 5.1732) (-10.9109, 5.1715) (-10.9204, 5.1694) (-10.9301, 5.1673) (-10.9383, 5.1654) (-10.9481, 5.1632) (-10.9578, 5.1609) (-10.9663, 5.1589) (-10.9762, 5.1565) (-10.9861, 5.154) (-10.9947, 5.1519) (-11.0048, 5.1493) (-11.0149, 5.1467) (-11.0236, 5.1444) (-11.0338, 5.1417) (-11.0441, 5.1389) (-11.0529, 5.1365) (-11.0633, 5.1336) (-11.0738, 5.1307) (-11.0827, 5.1281) (-11.0933, 5.125) (-11.1038, 5.1219) (-11.1129, 5.1192) (-11.1236, 5.116) (-11.1343, 5.1127) (-11.1436, 5.1098) (-11.1544, 5.1064) (-11.1652, 5.103) (-11.1746, 5.0999) (-11.1855, 5.0964) (-11.1965, 5.0927) (-11.206, 5.0895) (-11.217, 5.0858) (-11.2282, 5.082) (-11.2377, 5.0786) (-11.2489, 5.0747) (-11.2602, 5.0707) (-11.2699, 5.0672) (-11.2812, 5.0631) (-11.2925, 5.0589) (-11.3023, 5.0553) (-11.3138, 5.051) (-11.3252, 5.0466) (-11.3351, 5.0428) (-11.3467, 5.0383) (-11.3582, 5.0338) (-11.3682, 5.0298) (-11.3782, 5.0258) (-11.3932, 5.0197) (-11.4067, 5.0142) (-11.4201, 5.0086) (-11.4336, 5.0029) (-11.4506, 4.9957) (-11.4625, 4.9906) (-11.4744, 4.9854) (-11.4864, 4.9801) (-11.5018, 4.9732) (-11.5139, 4.9678) (-11.5259, 4.9623) (-11.5398, 4.9559) (-11.5537, 4.9495) (-11.5641, 4.9446) (-11.5745, 4.9396) (-11.585, 4.9346) (-11.5938, 4.9304) (-11.6025, 4.9262) (-11.6113, 4.9219) (-11.6201, 4.9176) (-11.6289, 4.9133) (-11.6377, 4.9089) (-11.6465, 4.9045) (-11.6553, 4.9) (-11.6642, 4.8956) (-11.673, 4.8911) (-11.6819, 4.8865) (-11.6908, 4.8819) (-11.6997, 4.8773) (-11.7086, 4.8726) (-11.7175, 4.8679) (-11.7265, 4.8632) (-11.7354, 4.8585) (-11.7444, 4.8537) (-11.7533, 4.8488) (-11.7623, 4.844) (-11.7713, 4.839) (-11.7803, 4.8341) (-11.7893, 4.8291) (-11.7983, 4.8241) (-11.8074, 4.8191) (-11.82, 4.812) (-11.8309, 4.8058) (-11.8399, 4.8006) (-11.8472, 4.7964) (-11.8527, 4.7933) knots 0 0 0 0 0 0 0.004167 0.008333 0.0125 0.016667 0.020833 0.025 0.029167 0.033333 0.0375 0.041667 0.045833 0.05 0.054167 0.058333 0.0625 0.066667 0.070833 0.075 0.079167 0.083333 0.0875 0.091667 0.095833 0.1 0.104167 0.108333 0.1125 0.116667 0.120833 0.125 0.129167 0.1375 0.141667 0.145833 0.154167 0.158333 0.1625 0.170833 0.175 0.179167 0.1875 0.191667 0.195833 0.204167 0.208333 0.2125 0.220833 0.225 0.229167 0.2375 0.241667 0.245833 0.254167 0.258333 0.2625 0.270833 0.275 0.279167 0.2875 0.291667 0.295833 0.304167 0.308333 0.3125 0.320833 0.325 0.329167 0.3375 0.341667 0.345833 0.354167 0.358333 0.3625 0.370833 0.375 0.379167 0.3875 0.391667 0.395833 0.404167 0.408333 0.4125 0.420833 0.425 0.429167 0.4375 0.441667 0.445833 0.454167 0.458333 0.4625 0.470833 0.475 0.479167 0.4875 0.491667 0.495833 0.504167 0.508333 0.5125 0.520833 0.525 0.529167 0.5375 0.541667 0.545833 0.554167 0.558333 0.5625 0.570833 0.575 0.579167 0.5875 0.591667 0.595833 0.604167 0.608333 0.6125 0.620833 0.625 0.629167 0.6375 0.641667 0.645833 0.654167 0.658333 0.6625 0.670833 0.675 0.679167 0.6875 0.691667 0.695833 0.704167 0.708333 0.7125 0.720833 0.725 0.729167 0.7375 0.741667 0.745833 0.754167 0.758333 0.7625 0.770833 0.775 0.779167 0.783333 0.8 0.804167 0.808333 0.8125 0.825 0.829167 0.833333 0.8375 0.85 0.854167 0.858333 0.866667 0.870833 0.875 0.879167 0.883333 0.8875 0.891667 0.895833 0.9 0.904167 0.908333 0.9125 0.916667 0.920833 0.925 0.929167 0.933333 0.9375 0.941667 0.945833 0.95 0.954167 0.958333 0.9625 0.966667 0.970833 0.975 0.979167 0.983333 0.9875 1 1 1 1 1 1
  line L10 (-10.5159, 3.5725) -> (-9.6305, 3.643)
  line L11 (-10.5165, 3.5724) -> (-10.5159, 3.5725)
  arc A5 (-11.8527, 4.7933) -> (-11.8938, 4.174) centre (-4.8955, 4.02) ccw
  spline S5 degree 5 poles (-11.8938, 4.174) (-11.8888, 4.1701) (-11.8822, 4.165) (-11.8739, 4.1587) (-11.8639, 4.1511) (-11.8523, 4.1424) (-11.844, 4.1362) (-11.8358, 4.1301) (-11.8275, 4.1239) (-11.8192, 4.1178) (-11.811, 4.1118) (-11.8027, 4.1058) (-11.7945, 4.0998) (-11.7862, 4.0939) (-11.778, 4.088) (-11.7698, 4.0821) (-11.7615, 4.0763) (-11.7533, 4.0705) (-11.7451, 4.0647) (-11.7369, 4.059) (-11.7287, 4.0533) (-11.7205, 4.0476) (-11.7123, 4.042) (-11.7042, 4.0365) (-11.696, 4.0309) (-11.6879, 4.0254) (-11.6797, 4.0199) (-11.6716, 4.0145) (-11.6634, 4.0091) (-11.6553, 4.0038) (-11.6456, 3.9974) (-11.6359, 3.9911) (-11.6262, 3.9848) (-11.6149, 3.9775) (-11.6036, 3.9703) (-11.5939, 3.9642) (-11.5843, 3.9582) (-11.5747, 3.9522) (-11.5651, 3.9462) (-11.5555, 3.9403) (-11.5459, 3.9345) (-11.5348, 3.9278) (-11.5236, 3.9211) (-11.5141, 3.9154) (-11.503, 3.9089) (-11.492, 3.9024) (-11.4825, 3.8969) (-11.4715, 3.8905) (-11.4606, 3.8843) (-11.4512, 3.8789) (-11.4402, 3.8728) (-11.4293, 3.8667) (-11.42, 3.8616) (-11.4076, 3.8548) (-11.3953, 3.8481) (-11.3845, 3.8423) (-11.3738, 3.8366) (-11.36, 3.8293) (-11.3493, 3.8237) (-11.3387, 3.8182) (-11.3281, 3.8128) (-11.3145, 3.8059) (-11.304, 3.8007) (-11.2935, 3.7955) (-11.2816, 3.7896) (-11.2697, 3.7839) (-11.2608, 3.7796) (-11.2504, 3.7747) (-11.2402, 3.7698) (-11.2314, 3.7657) (-11.2211, 3.761) (-11.211, 3.7563) (-11.2023, 3.7524) (-11.1922, 3.7478) (-11.1821, 3.7434) (-11.1735, 3.7396) (-11.1635, 3.7352) (-11.1536, 3.731) (-11.1451, 3.7274) (-11.1353, 3.7232) (-11.1255, 3.7191) (-11.1171, 3.7156) (-11.1074, 3.7117) (-11.0977, 3.7078) (-11.0895, 3.7045) (-11.0799, 3.7007) (-11.0704, 3.6969) (-11.0622, 3.6938) (-11.0528, 3.6902) (-11.0434, 3.6866) (-11.0354, 3.6837) (-11.0261, 3.6802) (-11.0169, 3.6769) (-11.0091, 3.674) (-10.9999, 3.6708) (-10.9909, 3.6676) (-10.9831, 3.6649) (-10.9742, 3.6618) (-10.9653, 3.6588) (-10.9577, 3.6563) (-10.9489, 3.6534) (-10.9401, 3.6505) (-10.9327, 3.6481) (-10.9241, 3.6454) (-10.9155, 3.6427) (-10.9082, 3.6405) (-10.8998, 3.6379) (-10.8914, 3.6354) (-10.8843, 3.6333) (-10.876, 3.6309) (-10.8678, 3.6286) (-10.8609, 3.6266) (-10.8528, 3.6244) (-10.8448, 3.6222) (-10.838, 3.6203) (-10.8301, 3.6183) (-10.8224, 3.6162) (-10.8157, 3.6145) (-10.8081, 3.6126) (-10.8005, 3.6107) (-10.7941, 3.6092) (-10.7866, 3.6074) (-10.7793, 3.6057) (-10.773, 3.6042) (-10.7658, 3.6026) (-10.7586, 3.601) (-10.7526, 3.5997) (-10.7456, 3.5982) (-10.7387, 3.5968) (-10.7328, 3.5956) (-10.7261, 3.5942) (-10.7194, 3.593) (-10.7137, 3.5919) (-10.7072, 3.5907) (-10.7008, 3.5895) (-10.6954, 3.5885) (-10.6891, 3.5874) (-10.6829, 3.5864) (-10.6777, 3.5856) (-10.6717, 3.5846) (-10.6658, 3.5837) (-10.6608, 3.5829) (-10.6551, 3.5821) (-10.6494, 3.5813) (-10.6447, 3.5806) (-10.6392, 3.5799) (-10.6339, 3.5792) (-10.6294, 3.5787) (-10.6242, 3.578) (-10.6191, 3.5775) (-10.6149, 3.577) (-10.61, 3.5765) (-10.6052, 3.576) (-10.6012, 3.5756) (-10.5973, 3.5752) (-10.5922, 3.5748) (-10.5878, 3.5744) (-10.583, 3.574) (-10.5783, 3.5737) (-10.5738, 3.5734) (-10.5705, 3.5732) (-10.5673, 3.573) (-10.5647, 3.5729) (-10.5621, 3.5727) (-10.5596, 3.5726) (-10.5572, 3.5725) (-10.5549, 3.5724) (-10.5526, 3.5723) (-10.5503, 3.5723) (-10.5481, 3.5722) (-10.546, 3.5722) (-10.544, 3.5721) (-10.542, 3.5721) (-10.5401, 3.572) (-10.5383, 3.572) (-10.5365, 3.572) (-10.5348, 3.572) (-10.5331, 3.572) (-10.5316, 3.572) (-10.5301, 3.572) (-10.5287, 3.572) (-10.5273, 3.572) (-10.526, 3.5721) (-10.5248, 3.5721) (-10.5237, 3.5721) (-10.5226, 3.5722) (-10.5216, 3.5722) (-10.5207, 3.5722) (-10.5199, 3.5723) (-10.5191, 3.5723) (-10.5184, 3.5723) (-10.5177, 3.5724) (-10.5172, 3.5724) (-10.5169, 3.5724) (-10.5166, 3.5724) (-10.5165, 3.5724) knots -1 -1 -1 -1 -1 -1 -0.9875 -0.983333 -0.979167 -0.975 -0.970833 -0.966667 -0.9625 -0.958333 -0.954167 -0.95 -0.945833 -0.941667 -0.9375 -0.933333 -0.929167 -0.925 -0.920833 -0.916667 -0.9125 -0.908333 -0.904167 -0.9 -0.895833 -0.891667 -0.8875 -0.883333 -0.879167 -0.875 -0.870833 -0.8625 -0.858333 -0.854167 -0.845833 -0.841667 -0.8375 -0.833333 -0.829167 -0.820833 -0.816667 -0.8125 -0.804167 -0.8 -0.795833 -0.7875 -0.783333 -0.779167 -0.770833 -0.766667 -0.7625 -0.754167 -0.75 -0.745833 -0.733333 -0.729167 -0.725 -0.720833 -0.708333 -0.704167 -0.7 -0.695833 -0.683333 -0.679167 -0.675 -0.666667 -0.6625 -0.658333 -0.65 -0.645833 -0.641667 -0.633333 -0.629167 -0.625 -0.616667 -0.6125 -0.608333 -0.6 -0.595833 -0.591667 -0.583333 -0.579167 -0.575 -0.566667 -0.5625 -0.558333 -0.55 -0.545833 -0.541667 -0.533333 -0.529167 -0.525 -0.516667 -0.5125 -0.508333 -0.5 -0.495833 -0.491667 -0.483333 -0.479167 -0.475 -0.466667 -0.4625 -0.458333 -0.45 -0.445833 -0.441667 -0.433333 -0.429167 -0.425 -0.416667 -0.4125 -0.408333 -0.4 -0.395833 -0.391667 -0.383333 -0.379167 -0.375 -0.366667 -0.3625 -0.358333 -0.35 -0.345833 -0.341667 -0.333333 -0.329167 -0.325 -0.316667 -0.3125 -0.308333 -0.3 -0.295833 -0.291667 -0.283333 -0.279167 -0.275 -0.266667 -0.2625 -0.258333 -0.25 -0.245833 -0.241667 -0.233333 -0.229167 -0.225 -0.216667 -0.2125 -0.208333 -0.2 -0.195833 -0.191667 -0.183333 -0.179167 -0.175 -0.170833 -0.158333 -0.154167 -0.145833 -0.141667 -0.1375 -0.133333 -0.129167 -0.125 -0.120833 -0.116667 -0.1125 -0.108333 -0.104167 -0.1 -0.095833 -0.091667 -0.0875 -0.083333 -0.079167 -0.075 -0.070833 -0.066667 -0.0625 -0.058333 -0.054167 -0.05 -0.045833 -0.041667 -0.0375 -0.033333 -0.029167 -0.025 -0.020833 -0.016667 -0.0125 -0.008333 0 0 0 0 0 0
  arc A6 (-9.6305, 3.643) -> (-9.417, 2.5644) centre (-4.8955, 4.02) ccw
  line L12 (-9.5397, 0.8219) -> (-9.5391, 0.8222)
  spline S6 degree 5 poles (-11.0332, 0.6542) (-11.027, 0.6533) (-11.0187, 0.6523) (-11.0083, 0.6509) (-10.9959, 0.6494) (-10.9815, 0.6476) (-10.9712, 0.6464) (-10.961, 0.6452) (-10.9508, 0.644) (-10.9406, 0.6429) (-10.9304, 0.6418) (-10.9202, 0.6407) (-10.9101, 0.6396) (-10.9, 0.6386) (-10.8899, 0.6376) (-10.8798, 0.6366) (-10.8698, 0.6357) (-10.8598, 0.6348) (-10.8498, 0.6339) (-10.8398, 0.6331) (-10.8299, 0.6322) (-10.82, 0.6314) (-10.8101, 0.6307) (-10.8002, 0.6299) (-10.7904, 0.6292) (-10.7806, 0.6285) (-10.7708, 0.6278) (-10.761, 0.6272) (-10.7513, 0.6266) (-10.7416, 0.626) (-10.73, 0.6254) (-10.7184, 0.6247) (-10.7068, 0.6242) (-10.6934, 0.6235) (-10.6801, 0.6229) (-10.6686, 0.6225) (-10.6573, 0.6221) (-10.6459, 0.6217) (-10.6346, 0.6213) (-10.6234, 0.621) (-10.6122, 0.6208) (-10.5992, 0.6205) (-10.5862, 0.6203) (-10.5751, 0.6201) (-10.5622, 0.62) (-10.5494, 0.6199) (-10.5385, 0.6199) (-10.5258, 0.6199) (-10.5131, 0.6199) (-10.5024, 0.62) (-10.488, 0.6202) (-10.4738, 0.6204) (-10.4614, 0.6206) (-10.449, 0.6209) (-10.4333, 0.6214) (-10.4211, 0.6218) (-10.4089, 0.6222) (-10.3969, 0.6227) (-10.3814, 0.6234) (-10.3695, 0.6239) (-10.3576, 0.6246) (-10.3458, 0.6252) (-10.3307, 0.6261) (-10.3191, 0.6269) (-10.3075, 0.6277) (-10.2943, 0.6286) (-10.2813, 0.6297) (-10.2715, 0.6305) (-10.2602, 0.6314) (-10.249, 0.6324) (-10.2394, 0.6333) (-10.2283, 0.6344) (-10.2172, 0.6355) (-10.2078, 0.6365) (-10.1969, 0.6376) (-10.186, 0.6388) (-10.1768, 0.6399) (-10.1661, 0.6412) (-10.1554, 0.6425) (-10.1464, 0.6436) (-10.1359, 0.645) (-10.1254, 0.6464) (-10.1166, 0.6476) (-10.1063, 0.6491) (-10.096, 0.6506) (-10.0873, 0.6519) (-10.0773, 0.6535) (-10.0673, 0.655) (-10.0587, 0.6564) (-10.0489, 0.658) (-10.0391, 0.6597) (-10.0308, 0.6611) (-10.0211, 0.6629) (-10.0116, 0.6646) (-10.0034, 0.6661) (-9.994, 0.6679) (-9.9847, 0.6697) (-9.9767, 0.6713) (-9.9675, 0.6731) (-9.9584, 0.675) (-9.9507, 0.6766) (-9.9417, 0.6785) (-9.9329, 0.6805) (-9.9253, 0.6821) (-9.9166, 0.6841) (-9.908, 0.6861) (-9.9007, 0.6878) (-9.8922, 0.6899) (-9.8838, 0.6919) (-9.8767, 0.6937) (-9.8685, 0.6957) (-9.8603, 0.6978) (-9.8534, 0.6996) (-9.8454, 0.7017) (-9.8375, 0.7038) (-9.8309, 0.7057) (-9.8231, 0.7078) (-9.8155, 0.71) (-9.809, 0.7118) (-9.8016, 0.714) (-9.7942, 0.7162) (-9.788, 0.7181) (-9.7807, 0.7202) (-9.7736, 0.7224) (-9.7676, 0.7243) (-9.7607, 0.7265) (-9.7538, 0.7287) (-9.7481, 0.7306) (-9.7414, 0.7328) (-9.7348, 0.7351) (-9.7293, 0.737) (-9.7229, 0.7392) (-9.7166, 0.7414) (-9.7113, 0.7433) (-9.7052, 0.7455) (-9.6992, 0.7477) (-9.6941, 0.7495) (-9.6883, 0.7517) (-9.6826, 0.7539) (-9.6777, 0.7557) (-9.6722, 0.7579) (-9.6668, 0.76) (-9.6622, 0.7619) (-9.657, 0.764) (-9.6518, 0.7661) (-9.6475, 0.7679) (-9.6426, 0.77) (-9.6378, 0.772) (-9.6337, 0.7738) (-9.6291, 0.7758) (-9.6245, 0.7778) (-9.6208, 0.7795) (-9.6164, 0.7814) (-9.6122, 0.7834) (-9.6087, 0.785) (-9.6047, 0.7869) (-9.6008, 0.7887) (-9.5975, 0.7903) (-9.5938, 0.7921) (-9.5903, 0.7938) (-9.5873, 0.7953) (-9.5844, 0.7968) (-9.5816, 0.7982) (-9.5793, 0.7993) (-9.5771, 0.8005) (-9.575, 0.8016) (-9.5729, 0.8027) (-9.5708, 0.8038) (-9.5689, 0.8048) (-9.5669, 0.8059) (-9.5651, 0.8069) (-9.5633, 0.8079) (-9.5616, 0.8088) (-9.5599, 0.8098) (-9.5583, 0.8107) (-9.5568, 0.8115) (-9.5553, 0.8124) (-9.5539, 0.8132) (-9.5525, 0.814) (-9.5512, 0.8147) (-9.55, 0.8155) (-9.5488, 0.8162) (-9.5477, 0.8168) (-9.5467, 0.8174) (-9.5457, 0.818) (-9.5448, 0.8186) (-9.544, 0.8191) (-9.5432, 0.8196) (-9.5425, 0.8201) (-9.5418, 0.8205) (-9.5413, 0.8208) (-9.5406, 0.8212) (-9.5402, 0.8215) (-9.5399, 0.8217) (-9.5398, 0.8218) (-9.5397, 0.8219) knots -1 -1 -1 -1 -1 -1 -0.9875 -0.983333 -0.979167 -0.975 -0.970833 -0.966667 -0.9625 -0.958333 -0.954167 -0.95 -0.945833 -0.941667 -0.9375 -0.933333 -0.929167 -0.925 -0.920833 -0.916667 -0.9125 -0.908333 -0.904167 -0.9 -0.895833 -0.891667 -0.8875 -0.883333 -0.879167 -0.875 -0.870833 -0.8625 -0.858333 -0.854167 -0.845833 -0.841667 -0.8375 -0.833333 -0.829167 -0.820833 -0.816667 -0.8125 -0.804167 -0.8 -0.795833 -0.7875 -0.783333 -0.779167 -0.770833 -0.766667 -0.7625 -0.75 -0.745833 -0.741667 -0.7375 -0.725 -0.720833 -0.716667 -0.7125 -0.7 -0.695833 -0.691667 -0.6875 -0.675 -0.670833 -0.666667 -0.658333 -0.654167 -0.65 -0.641667 -0.6375 -0.633333 -0.625 -0.620833 -0.616667 -0.608333 -0.604167 -0.6 -0.591667 -0.5875 -0.583333 -0.575 -0.570833 -0.566667 -0.558333 -0.554167 -0.55 -0.541667 -0.5375 -0.533333 -0.525 -0.520833 -0.516667 -0.508333 -0.504167 -0.5 -0.491667 -0.4875 -0.483333 -0.475 -0.470833 -0.466667 -0.458333 -0.454167 -0.45 -0.441667 -0.4375 -0.433333 -0.425 -0.420833 -0.416667 -0.408333 -0.404167 -0.4 -0.391667 -0.3875 -0.383333 -0.375 -0.370833 -0.366667 -0.358333 -0.354167 -0.35 -0.341667 -0.3375 -0.333333 -0.325 -0.320833 -0.316667 -0.308333 -0.304167 -0.3 -0.291667 -0.2875 -0.283333 -0.275 -0.270833 -0.266667 -0.258333 -0.254167 -0.25 -0.241667 -0.2375 -0.233333 -0.225 -0.220833 -0.216667 -0.208333 -0.204167 -0.2 -0.191667 -0.1875 -0.183333 -0.175 -0.170833 -0.166667 -0.158333 -0.154167 -0.15 -0.141667 -0.1375 -0.133333 -0.129167 -0.125 -0.120833 -0.116667 -0.1125 -0.108333 -0.104167 -0.1 -0.095833 -0.091667 -0.0875 -0.083333 -0.079167 -0.075 -0.070833 -0.066667 -0.0625 -0.058333 -0.054167 -0.05 -0.045833 -0.041667 -0.0375 -0.033333 -0.029167 -0.025 -0.020833 -0.016667 -0.0125 -0.008333 0 0 0 0 0 0
  line L13 (-9.5391, 0.8222) -> (-8.8076, 1.326)
  arc A7 (-8.8076, 1.326) -> (-8.0834, 0.4987) centre (-4.8955, 4.02) ccw
  line L14 (-8.6795, -0.1597) -> (-8.6799, -0.1602)
  line L15 (-8.0834, 0.4987) -> (-8.6795, -0.1597)
  spline S7 degree 5 poles (-8.6799, -0.1602) (-8.68, -0.1603) (-8.6801, -0.1604) (-8.6802, -0.1605) (-8.6805, -0.1608) (-8.6808, -0.1612) (-8.6812, -0.1617) (-8.6816, -0.1622) (-8.6821, -0.1628) (-8.6827, -0.1634) (-8.6832, -0.1641) (-8.6839, -0.1649) (-8.6845, -0.1657) (-8.6853, -0.1666) (-8.686, -0.1675) (-8.6868, -0.1685) (-8.6877, -0.1696) (-8.6885, -0.1707) (-8.6895, -0.1719) (-8.6904, -0.1731) (-8.6914, -0.1744) (-8.6925, -0.1758) (-8.6935, -0.1772) (-8.6946, -0.1787) (-8.6958, -0.1802) (-8.697, -0.1818) (-8.6982, -0.1834) (-8.6994, -0.1851) (-8.7007, -0.1869) (-8.702, -0.1887) (-8.7033, -0.1906) (-8.7047, -0.1925) (-8.7064, -0.1949) (-8.7081, -0.1974) (-8.7099, -0.1999) (-8.712, -0.203) (-8.7141, -0.2062) (-8.716, -0.209) (-8.7183, -0.2124) (-8.7206, -0.2159) (-8.7226, -0.219) (-8.7246, -0.2222) (-8.727, -0.2259) (-8.7302, -0.2309) (-8.7334, -0.2361) (-8.7367, -0.2415) (-8.7401, -0.2471) (-8.7435, -0.2528) (-8.7462, -0.2573) (-8.7489, -0.262) (-8.7517, -0.2668) (-8.7548, -0.2723) (-8.7577, -0.2773) (-8.7601, -0.2817) (-8.7629, -0.2868) (-8.7658, -0.2921) (-8.7683, -0.2967) (-8.7712, -0.3022) (-8.7742, -0.3077) (-8.7767, -0.3125) (-8.7797, -0.3183) (-8.7827, -0.3241) (-8.7853, -0.3292) (-8.7883, -0.3352) (-8.7914, -0.3413) (-8.794, -0.3466) (-8.7971, -0.3529) (-8.8002, -0.3593) (-8.8028, -0.3648) (-8.8059, -0.3714) (-8.809, -0.378) (-8.8117, -0.3838) (-8.8148, -0.3906) (-8.8179, -0.3975) (-8.8206, -0.4035) (-8.8238, -0.4106) (-8.8269, -0.4178) (-8.8296, -0.424) (-8.8328, -0.4314) (-8.8359, -0.4388) (-8.8386, -0.4452) (-8.8418, -0.4528) (-8.8449, -0.4605) (-8.8476, -0.4672) (-8.8507, -0.4751) (-8.8539, -0.483) (-8.8566, -0.4899) (-8.8597, -0.498) (-8.8628, -0.5062) (-8.8655, -0.5133) (-8.8686, -0.5216) (-8.8717, -0.5301) (-8.8743, -0.5374) (-8.8774, -0.5459) (-8.8805, -0.5546) (-8.8831, -0.5621) (-8.8862, -0.571) (-8.8892, -0.5799) (-8.8918, -0.5876) (-8.8949, -0.5967) (-8.8979, -0.6058) (-8.9004, -0.6138) (-8.9034, -0.6231) (-8.9064, -0.6324) (-8.9089, -0.6406) (-8.9118, -0.6501) (-8.9147, -0.6597) (-8.9172, -0.668) (-8.9201, -0.6778) (-8.9229, -0.6876) (-8.9254, -0.6961) (-8.9282, -0.7061) (-8.931, -0.7162) (-8.9334, -0.7249) (-8.9361, -0.7351) (-8.9388, -0.7454) (-8.9412, -0.7543) (-8.9439, -0.7647) (-8.9465, -0.7752) (-8.9488, -0.7843) (-8.9514, -0.7949) (-8.954, -0.8056) (-8.9562, -0.8149) (-8.9587, -0.8257) (-8.9612, -0.8367) (-8.9634, -0.8461) (-8.9658, -0.8571) (-8.9682, -0.8683) (-8.9703, -0.8779) (-8.9727, -0.8891) (-8.975, -0.9005) (-8.977, -0.9103) (-8.9793, -0.9217) (-8.9815, -0.9333) (-8.9834, -0.9432) (-8.9856, -0.9549) (-8.9878, -0.9666) (-8.9896, -0.9768) (-8.9917, -0.9886) (-8.9938, -1.0006) (-8.9955, -1.0108) (-8.9975, -1.0229) (-8.9995, -1.035) (-9.0011, -1.0455) (-9.003, -1.0577) (-9.0048, -1.07) (-9.0064, -1.0806) (-9.0084, -1.0948) (-9.0104, -1.1091) (-9.0121, -1.1217) (-9.0138, -1.1344) (-9.0154, -1.1471) (-9.0172, -1.1617) (-9.0189, -1.1764) (-9.0206, -1.1911) (-9.0222, -1.206) (-9.024, -1.2228) (-9.0251, -1.234) (-9.0262, -1.2453) (-9.0277, -1.2605) (-9.029, -1.2757) (-9.0302, -1.289) (-9.0313, -1.3025) (-9.0324, -1.316) (-9.0331, -1.3257) (-9.0338, -1.3354) (-9.0345, -1.3451) (-9.0352, -1.3548) (-9.0358, -1.3646) (-9.0364, -1.3745) (-9.037, -1.3843) (-9.0376, -1.3942) (-9.0381, -1.4041) (-9.0386, -1.414) (-9.0391, -1.424) (-9.0396, -1.434) (-9.0401, -1.444) (-9.0405, -1.454) (-9.0409, -1.4641) (-9.0412, -1.4742) (-9.0416, -1.4843) (-9.0419, -1.4945) (-9.0422, -1.5047) (-9.0425, -1.5149) (-9.0427, -1.5251) (-9.043, -1.5354) (-9.0431, -1.5457) (-9.0433, -1.556) (-9.0435, -1.5663) (-9.0436, -1.5808) (-9.0437, -1.5933) (-9.0438, -1.6038) (-9.0438, -1.6121) (-9.0438, -1.6184) knots 0 0 0 0 0 0 0.004167 0.008333 0.0125 0.016667 0.020833 0.025 0.029167 0.033333 0.0375 0.041667 0.045833 0.05 0.054167 0.058333 0.0625 0.066667 0.070833 0.075 0.079167 0.083333 0.0875 0.091667 0.095833 0.1 0.104167 0.108333 0.1125 0.116667 0.120833 0.125 0.129167 0.1375 0.141667 0.145833 0.154167 0.158333 0.1625 0.170833 0.175 0.179167 0.183333 0.191667 0.208333 0.2125 0.216667 0.220833 0.229167 0.2375 0.241667 0.245833 0.254167 0.258333 0.2625 0.270833 0.275 0.279167 0.2875 0.291667 0.295833 0.304167 0.308333 0.3125 0.320833 0.325 0.329167 0.3375 0.341667 0.345833 0.354167 0.358333 0.3625 0.370833 0.375 0.379167 0.3875 0.391667 0.395833 0.404167 0.408333 0.4125 0.420833 0.425 0.429167 0.4375 0.441667 0.445833 0.454167 0.458333 0.4625 0.470833 0.475 0.479167 0.4875 0.491667 0.495833 0.504167 0.508333 0.5125 0.520833 0.525 0.529167 0.5375 0.541667 0.545833 0.554167 0.558333 0.5625 0.570833 0.575 0.579167 0.5875 0.591667 0.595833 0.604167 0.608333 0.6125 0.620833 0.625 0.629167 0.6375 0.641667 0.645833 0.654167 0.658333 0.6625 0.670833 0.675 0.679167 0.6875 0.691667 0.695833 0.704167 0.708333 0.7125 0.720833 0.725 0.729167 0.7375 0.741667 0.745833 0.754167 0.758333 0.7625 0.770833 0.775 0.779167 0.791667 0.795833 0.8 0.804167 0.808333 0.825 0.829167 0.833333 0.8375 0.845833 0.85 0.854167 0.866667 0.870833 0.875 0.879167 0.883333 0.8875 0.891667 0.895833 0.9 0.904167 0.908333 0.9125 0.916667 0.920833 0.925 0.929167 0.933333 0.9375 0.941667 0.945833 0.95 0.954167 0.958333 0.9625 0.966667 0.970833 0.975 0.979167 0.983333 0.9875 1 1 1 1 1 1
  arc A8 (-9.0438, -1.6184) -> (-8.528, -1.9637) centre (-4.8955, 4.02) ccw
  line L16 (-7.3184, -1.0717) -> (-7.3181, -1.0712)
  line L17 (-7.3181, -1.0712) -> (-6.9365, -0.2692)
  arc A9 (-6.9365, -0.2692) -> (-5.8957, -0.6235) centre (-4.8955, 4.02) ccw